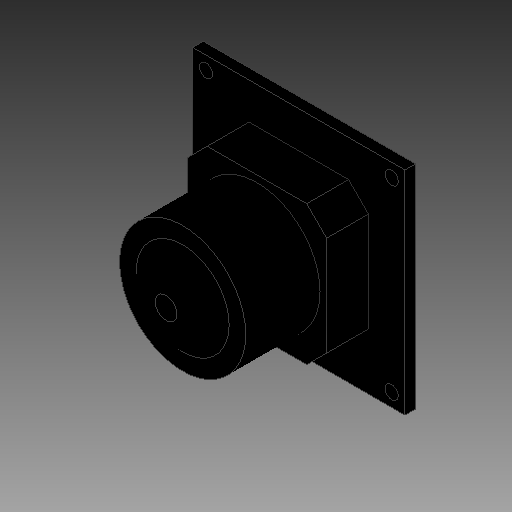
# Autodesk Inventor part: 超広角カメラ_MCM-4350FISH
Saved by Autodesk Inventor 2017 (Build 210142000, 142)
## iProperties
Created: 2016-08-22
Part Number: 超広角カメラ_MCM-4350FISH
Material: 一般
Document SubType Name: Modeling
Designer: NN
Density: 1 g/cm^3
Appearance: 陽極酸化 - 黒
Mass: 7.83753 g
Surface Area: 35.7184 cm^2
Volume: 7.83753 cm^3
Author: NN
Autodesk Inventor part; units mm, degrees
ref_plane "YZ Plane" through (0, 0, 0) normal (1, 0, 0) x (0, 1, 0)
ref_plane "XZ Plane" through (0, 0, 0) normal (0, 1, 0) x (-1, 0, 0)
ref_plane "XY Plane" through (0, 0, 0) normal (0, 0, 1) x (1, 0, 0)
sketch "スケッチ1" plane through (0, 0, 0) normal (0, 0, 1) x (1, 0, 0)
  line L0 (0, 0) -> (32, 0)
  line L1 (32, 0) -> (32, 32)
  line L2 (32, 32) -> (0, 32)
  line L3 (0, 32) -> (0, 0)
  dimension "d0" = 32
  dimension "d1" = 32
  constraints: 8 end point, 2 parallel, 1 horizontal, 1 perpendicular
  measures "d0" distance of L0.start L0.end
  measures "d1" distance of L2.end L0.start
extrude "押し出し1" add sketch "スケッチ1" along normal blind 1.6
sketch "スケッチ2" plane through (0, 0, 1.6) normal (0, 0, 1) x (1, 0, 0)
  line L0 (0, 0) -> (32, 0) projected
  line L1 (32, 0) -> (32, 32) projected
  line L2 (32, 32) -> (0, 32) projected
  line L3 (0, 32) -> (0, 0) projected
  line L4 (30, 2) -> (2, 2)
  line L5 (2, 2) -> (2, 30)
  line L6 (2, 30) -> (30, 30)
  line L7 (30, 30) -> (30, 2)
  dimension "d4" = 28
  constraints: 8 end point, 3 other
  measures "d4" distance of L4.start L4.end
hole "穴1" at (30, 30, 1.6) at (30, 2, 1.6) at (2, 2, 1.6) at (2, 30, 1.6) direction (0, 0, -1) diameter 2 end through all
sketch "スケッチ3" plane through (0, 0, 1.6) normal (0, 0, 1) x (1, 0, 0)
  line L0 (5.5, 26.5) -> (26.5, 26.5)
  line L1 (26.5, 26.5) -> (26.5, 5.5)
  line L2 (26.5, 5.5) -> (5.5, 5.5)
  line L3 (5.5, 5.5) -> (5.5, 26.5)
  circle A0 centre (2, 2) radius 1 projected
  circle A1 centre (30, 30) radius 1 projected
  circle A2 centre (30, 2) radius 1 projected
  circle A3 centre (2, 30) radius 1 projected
  line L4 (0, 0) -> (32, 0) projected
  line L5 (32, 0) -> (32, 32) projected
  line L6 (32, 32) -> (0, 32) projected
  line L7 (0, 32) -> (0, 0) projected
  line L8 (16, 26.5) -> (16, 32)
  line L9 (32, 32) -> (0, 32) projected
  line L10 (5.5, 16) -> (0, 16)
  line L11 (0, 32) -> (0, 0) projected
  dimension "d12" = 21
  dimension "d13" = 21
  constraints: 12 end point, 4 midpoint, 3 perpendicular, 2 parallel, 1 horizontal
  measures "d12" distance of L0.start L0.end
  measures "d13" distance of L2.end L0.start
extrude "押し出し2" add sketch "スケッチ3" along normal blind 6.3 contours L0 L1 L2 L3
sketch "スケッチ4" plane through (0, 0, 7.9) normal (0, 0, 1) x (1, 0, 0)
  line L0 (5.5, 26.5) -> (5.5, 5.5) projected
  line L1 (5.5, 5.5) -> (26.5, 5.5) projected
  line L2 (26.5, 5.5) -> (26.5, 26.5) projected
  line L3 (26.5, 26.5) -> (5.5, 26.5) projected
  line L4 (5.5, 26.5) -> (26.5, 26.5) projected
  line L5 (16, 26.5) -> (16, 5.5)
  line L6 (5.5, 5.5) -> (26.5, 5.5) projected
  circle A0 centre (16, 16) radius 9.5
  point P0 (0, 0)
  dimension "d16" = 19
  constraints: 3 midpoint, 2 end point, 1 centre point
  measures "d16" diameter of A0
extrude "押し出し3" add sketch "スケッチ4" along normal blind 11.2 contours A0 L5 | L5 A0
sketch "スケッチ5" plane through (16, 16, 19.1) normal (0, 0, 1) x (1, 0, 0)
  circle A0 centre (0, 0) radius 9.5 projected
  circle A1 centre (0, 0) radius 7
  point P0 (-16, -16)
  dimension "d19" = 14
  constraints: 1 centre point, 1 coincident
  measures "d19" diameter of A1
extrude "押し出し4" add sketch "スケッチ5" along normal blind 2.5 contours A1
fillet "フィレット1" radius 7 1 edges at (9, 16, 21.6)
sketch "スケッチ6" plane through (0, 0, 0) normal (0, 0, -1) x (-1, 0, 0)
  line L0 (-14, 4.1) -> (-6, 4.1)
  line L1 (-6, 4.1) -> (-6, 0.9)
  line L2 (-6, 0.9) -> (-14, 0.9)
  line L3 (-14, 0.9) -> (-14, 4.1)
  line L4 (0, 0) -> (-32, 0) projected
  line L5 (0, 32) -> (0, 0) projected
  dimension "d23" = 8
  dimension "d24" = 3.2
  dimension "d25" = 4.1
  dimension "d26" = 14
  constraints: 8 end point, 2 parallel, 1 horizontal, 1 perpendicular
  measures "d23" distance between parallel lines of L1 L3
  measures "d24" distance between parallel lines of L0 L2
  measures "d25" distance between parallel lines of L4 L0
  measures "d26" distance between parallel lines of L5 L3
extrude "押し出し5" add sketch "スケッチ6" along normal blind 5.5
chamfer "面取り1" distance 3 angle 45 4 edges at (5.5, 5.5, 4.75) (26.5, 5.5, 4.75) (26.5, 26.5, 4.75) (5.5, 26.5, 4.75)
